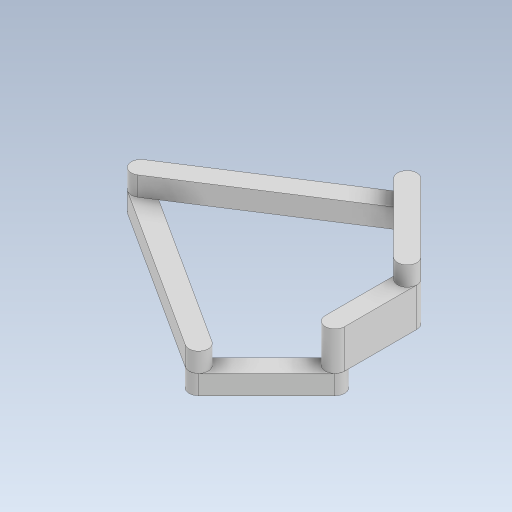
# Autodesk Inventor part: 5 Barras Simplificado
Saved by Autodesk Inventor 2024.2 (Build 282272000, 272)
## iProperties
Created: 2024-02-01
Part Number: 5 Barras Simplificado
Material: Generic
Document SubType Name: Modeling
Designer: juanp
Density: 1 g/cm^3
Appearance: Default
Author: juanp
Autodesk Inventor part; units mm, degrees
ref_plane "YZ Plane" through (0, 0, 0) normal (1, 0, 0) x (0, 1, 0)
ref_plane "XZ Plane" through (0, 0, 0) normal (0, 1, 0) x (-1, 0, 0)
ref_plane "XY Plane" through (0, 0, 0) normal (0, 0, 1) x (1, 0, 0)
sketch "Sketch1" plane through (0, 0, 0) normal (0, 1, 0) x (-1, 0, 0)
  line L0 (1000, 500) -> (0, 500) construction
  line L1 (0, 500) -> (0, -500) construction
  line L2 (0, -500) -> (1000, -500) construction
  line L3 (1000, -500) -> (1000, 500) construction
  line L4 (0, 37.5) -> (0, -37.5) construction
  line L5 (10, 37.5) -> (10, -37.5)
  line L6 (-10, -37.5) -> (-10, 37.5)
  arc A0 (10, 37.5) -> (-10, 37.5) centre (0, 37.5) ccw
  arc A1 (-10, -37.5) -> (10, -37.5) centre (0, -37.5) ccw
  line L7 (70.7107, 108.2107) -> (0, 37.5) construction
  line L8 (63.6396, 115.2817) -> (-7.0711, 44.5711)
  line L9 (7.0711, 30.4289) -> (77.7817, 101.1396)
  arc A2 (77.7817, 101.1396) -> (63.6396, 115.2817) centre (70.7107, 108.2107) ccw
  arc A3 (-7.0711, 44.5711) -> (7.0711, 30.4289) centre (0, 37.5) ccw
  line L10 (70.7107, -108.2107) -> (0, -37.5) construction
  line L11 (77.7817, -101.1396) -> (7.0711, -30.4289)
  line L12 (-7.0711, -44.5711) -> (63.6396, -115.2817)
  arc A4 (63.6396, -115.2817) -> (77.7817, -101.1396) centre (70.7107, -108.2107) ccw
  arc A5 (7.0711, -30.4289) -> (-7.0711, -44.5711) centre (0, -37.5) ccw
  line L13 (70.7107, 108.2107) -> (238.9083, 0) construction
  line L14 (76.1212, 116.6206) -> (244.3189, 8.4099)
  line L15 (233.4978, -8.4099) -> (65.3001, 99.8008)
  arc A6 (76.1212, 116.6206) -> (65.3001, 99.8008) centre (70.7107, 108.2107) ccw
  arc A7 (233.4978, -8.4099) -> (244.3189, 8.4099) centre (238.9083, 0) ccw
  line L16 (70.7107, -108.2107) -> (238.9083, 0) construction
  line L17 (76.1212, -116.6206) -> (244.3189, -8.4099)
  line L18 (233.4978, 8.4099) -> (65.3001, -99.8008)
  arc A8 (65.3001, -99.8008) -> (76.1212, -116.6206) centre (70.7107, -108.2107) ccw
  arc A9 (244.3189, -8.4099) -> (233.4978, 8.4099) centre (238.9083, 0) ccw
  line L19 (70.7107, -108.2107) -> (70.7107, -536.9645) construction
  line L20 (70.7107, 108.2107) -> (70.7107, -95.8947) construction
  point P0 (0, 0)
  point P1 (0, 0)
  point P2 (0, 0)
  point P3 (35.3553, 72.8553)
  point P4 (35.3553, -72.8553)
  point P5 (154.8095, 54.1053)
  point P6 (154.8095, -54.1053)
  point P7 (-7.0711, 44.5711)
  point P8 (-10, 37.5)
  point P9 (63.6396, -115.2817)
  point P10 (76.1212, -116.6206)
  point P11 (244.3189, -8.4099)
  point P12 (244.3189, 8.4099)
  point P13 (76.1212, 116.6206)
  point P14 (63.6396, 115.2817)
  point P15 (-7.0711, -44.5711)
  dimension "d42" = 1000
  dimension "d43" = 1000
  dimension "d45" = 75
  dimension "d46" = 20
  dimension "d47" = 20
  dimension "d48" = 20
  dimension "d49" = 20
  dimension "d50" = 20
  dimension "d51" = 100
  dimension "d52" = 100
  dimension "d53" = 200
  dimension "d54" = 200
  dimension "d55" = 45
  dimension "d56" = 45
  dimension "d71" = 122.755
  dimension "d72" = 57.245
  dimension "d73" = 154.8095
  dimension "d74" = 54.1053
  dimension "d75" = 35.3553
  dimension "d76" = 72.8553
  dimension "d77" = 77.755
  dimension "d78" = 37.5
  dimension "d79" = 35.36
  constraints: 52 end point, 20 point on circle, 20 tangent, 10 centre point, 7 parallel, 6 midpoint, 3 vertical, 2 coincident, 1 horizontal, 1 perpendicular
  measures "d42" distance of L2.end L1.end
  measures "d43" distance of L2.end L0.start
  measures "d45" distance of L4.start L4.end
  measures "d46" distance between parallel lines of L5 L6
  measures "d47" distance between parallel lines of L14 L15
  measures "d48" distance between parallel lines of L17 L18
  measures "d49" distance between parallel lines of L9 L8
  measures "d50" distance between parallel lines of L12 L11
  measures "d51" distance of L4.start L7.start
  measures "d52" distance of L4.end L10.start
  measures "d53" distance of L13.end L7.start
  measures "d54" distance of L10.start L13.end
  measures "d55" angle of L10 L4
  measures "d56" angle of L7 L1
  measures "d71" angle of L16 L19
  measures "d72" angle of L13 L20
  measures "d73" distance from line of point (154.81, -54.105) L1
  measures "d74" vertical distance of point (154.81, -54.105) point (0, 0)
  measures "d75" horizontal distance of point (35.355, -72.855) point (0, 0)
  measures "d76" vertical distance of point (35.355, -72.855) point (0, 0)
  measures "d77" angle of L13 L7
  measures "d78" distance of L4.start point (0, 0)
extrude "Extrusion6" add sketch "Sketch1" against normal blind 20 contours A0 L8 A6 L15 L9 L5 | L5 L9 A3 A0 | L15 A6 A2 L9
extrude "Extrusion7" add sketch "Sketch1" along normal blind 20 separate body contours L15 A6 A2 L9 | L9 A2 L14 A9 L18 L15 | L18 A9 A7 L15
extrude "Extrusion8" add sketch "Sketch1" along normal blind 40 separate body contours L18 L15 A7 L17 A4 L11 | L11 A4 A8 L18 | L18 A9 A7 L15
extrude "Extrusion9" add sketch "Sketch1" along normal blind 60 separate body contours L11 L18 A8 L12 A1 L5 | L5 A1 A5 L11 | L11 A4 A8 L18
extrude "Extrusion10" cut sketch "Sketch1" along normal blind 20 contours L18 L15 A7 L17 A4 L11 | L11 A4 A8 L18 | L18 A9 A7 L15 bodies 3
extrude "Extrusion11" cut sketch "Sketch1" along normal blind 40 contours L11 L18 A8 L12 A1 L5 | L5 A1 A5 L11 | L11 A4 A8 L18 bodies 4
extrude "Extrusion12" add sketch "Sketch1" along normal blind 40 separate body contours L5 L9 A3 A0 | L5 L11 A5 L6 A3 L9 | L5 A1 A5 L11
equation "\"d45\" = L_G"
equation "\"d46\" = t"
equation "\"d47\" = t"
equation "\"d48\" = t"
equation "\"d49\" = t"
equation "\"d50\" = t"
equation "\"d51\" = L_P"
equation "\"d52\" = L_P"
equation "\"d53\" = L_D"
equation "\"d54\" = L_D"
equation "\"d57\" = t"
equation "\"d59\" = t"
equation "\"d61\" = 2 * t"
equation "\"d63\" = 3 * t"
equation "\"d65\" = t"
equation "\"d67\" = 2 * t"
equation "\"d69\" = 2 * t"
equation "\"L_G\" = 150 * scale"
equation "\"L_P\" = 200 * scale"
equation "\"L_D\" = 400 * scale"
equation "\"t\" = 40 * scale"
equation "\"scale\" = 0.5"
body "Solid6"
body "Solid7"
body "Solid8"
body "Solid9"
body "Solid10"
